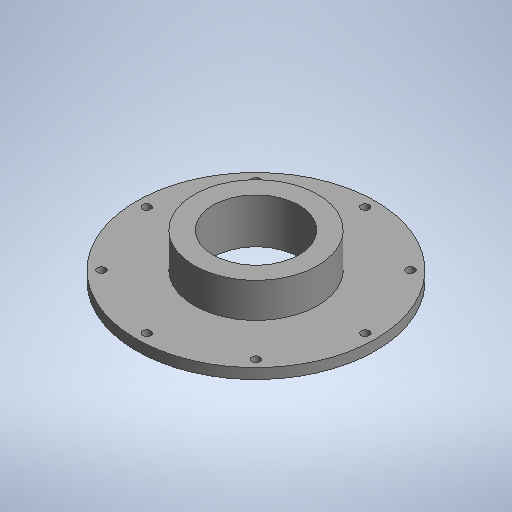
# Autodesk Inventor part: DMF Hat 2.0
Saved by Autodesk Inventor 2025 (Build 290162010, 162A)
## iProperties
Part Number: DMF Hat 2.0
Material: Generic
Document SubType Name: Modeling
Designer: pokla
Appearance: Default
Author: pokla
Autodesk Inventor part; units mm, degrees
ref_plane "YZ Plane" through (0, 0, 0) normal (1, 0, 0) x (0, 1, 0)
ref_plane "XZ Plane" through (0, 0, 0) normal (0, 1, 0) x (-1, 0, 0)
ref_plane "XY Plane" through (0, 0, 0) normal (0, 0, 1) x (1, 0, 0)
sketch "Sketch2" plane through (0, 0, 0) normal (0, 0, 1) x (1, 0, 0)
  line L0 (67, 70) -> (67, 0)
  line L1 (67, 0) -> (186, 0)
  line L2 (186, 0) -> (186, 16)
  line L3 (186, 16) -> (96, 16)
  line L4 (96, 16) -> (96, 70)
  line L5 (96, 70) -> (67, 70)
  line L6 (0, 0) -> (0, 134.3394)
  dimension "d1" = 70
  dimension "d2" = 119
  dimension "d3" = 29
  dimension "d4" = 134
  dimension "d5" = 16
  constraints: 14 end point, 5 perpendicular, 2 vertical, 1 horizontal alignment
  measures "d1" distance between parallel lines of L1 L5
  measures "d2" distance of L0.end L1.end
  measures "d3" distance of L4.end L0.start
  measures "d4" diameter of L0 L6
  measures "d5" distance between parallel lines of L1 L3
revolve "Revolution1" add sketch "Sketch2" angle 360 about axis through (0, 0, 0) along (0, 1, 0)
sketch "Sketch3" plane through (0, 16, 0) normal (0, 1, 0) x (1, 0, 0)
  circle A0 centre (0, 0) radius 170 construction
  point P0 (0, 170)
  dimension "d7" = 340
  constraints: 2 vertical alignment, 1 coincident, 2 other
hole "Hole1" at (0, 16, -170) direction (0, -1, 0) diameter 13 end through all
pattern_circular "Circular Pattern1" count 8 over 360 about axis through (0, -10, 0) along (0, 1, 0) of "Hole1"
body "Solid1"
